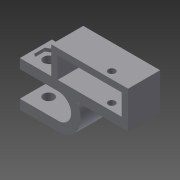
# Autodesk Inventor part: EndStopClip8mm
Saved by Autodesk Inventor 2014 SP1 (Build 180222100, 222)
## iProperties
Created: 2014-03-02
Part Number: EndStopClip8mm
Material: Generic
Document SubType Name: Modeling
Designer: Jack
Density: 1 g/cm^3
Appearance: Default
Author: Jack
Autodesk Inventor part; units mm, degrees
ref_plane "YZ Plane" through (0, 0, 0) normal (1, 0, 0) x (0, 1, 0)
ref_plane "XZ Plane" through (0, 0, 0) normal (0, 1, 0) x (-1, 0, 0)
ref_plane "XY Plane" through (0, 0, 0) normal (0, 0, 1) x (1, 0, 0)
sketch "Sketch1" plane through (0, 0, 0) normal (0, 1, 0) x (-1, 0, 0)
  arc A0 (0, 4) -> (0, -4) centre (0, 0) ccw
  line L0 (-19.8, 7.6035) -> (0, 7.6035) construction
  line L1 (0, 7.6035) -> (0, 14.0035) construction
  line L2 (0, 14.0035) -> (-19.8, 14.0035) construction
  line L3 (-19.8, 14.0035) -> (-19.8, 7.6035) construction
  line L4 (0, 7) -> (-21.8, 7)
  line L5 (0, 7) -> (12, 7)
  line L6 (12, 7) -> (12, 4)
  line L7 (12, 4) -> (5.7446, 4)
  line L8 (0, -7) -> (12, -7)
  line L9 (12, -7) -> (12, -4)
  line L10 (12, -4) -> (5.7446, -4)
  line L11 (-5.7446, 4) -> (-21.8, 4)
  line L12 (-21.8, 4) -> (-21.8, 7)
  line L13 (5.7446, 4) -> (0, 4)
  line L14 (5.7446, -4) -> (0, -4)
  arc A1 (-5.7446, 4) -> (0, -7) centre (0, 0) ccw
  dimension "d0" = 8
  dimension "d1" = 19.8
  dimension "d2" = 6.4
  dimension "d3" = 19.8
  dimension "d5" = 21.8
  dimension "d6" = 12
  dimension "d7" = 3
  dimension "d8" = 3
  dimension "d9" = 3
  dimension "d10" = 12
  dimension "d11" = 7
  dimension "d12" = 7
  dimension "d13" = 21.8
  constraints: 30 end point, 7 perpendicular, 5 parallel, 4 point on circle, 2 centre point, 2 coincident, 1 collinear, 1 horizontal, 1 tangent, 1 vertical alignment
  measures "d0" diameter of A0
  measures "d1" distance of L0.start L0.end
  measures "d2" distance of L0.end L1.end
  measures "d3" distance of L1.end L2.end
  measures "d5" distance of L4.start L4.end
  measures "d6" distance of L4.start L5.end
  measures "d7" distance of L5.end L6.end
  measures "d8" distance of L8.end L9.end
  measures "d9" distance of L11.end L4.end
  measures "d10" distance of L8.start L8.end
  measures "d11" radius of A1
  measures "d12" distance from line of point (0, 0) L4
  measures "d13" distance from line of L12 point (0, 0)
extrude "Extrusion1" add sketch "Sketch1" along normal blind 10
sketch "Sketch2" plane through (0, 0, -7) normal (0, 0, -1) x (-1, 0, 0)
  line L0 (12, 0) -> (12, 10) projected
  line L1 (0, 10) -> (12, 10) projected
  circle A0 centre (8, 5) radius 1.65
  dimension "d16" = 3.3
  dimension "d17" = 4
  dimension "d18" = 5
  constraints: 1 centre point
  measures "d16" diameter of A0
  measures "d17" distance from line of L0 A0.centre
  measures "d18" distance from line of L1 A0.centre
extrude "Extrusion2" cut sketch "Sketch2" against normal up to surface (14 mm away)
sketch "Sketch3" plane through (-12, 0, 7) normal (0, 0, 1) x (1, 0, 0)
  line L0 (0, 0) -> (33.8, 0) projected
  line L1 (33.8, 0) -> (33.8, 10) projected
  line L2 (0, 10) -> (33.8, 10) projected
  line L3 (31.8, 10) -> (31.8, 0)
  point P0 (12, 0)
  dimension "d21" = 2
  constraints: 2 end point, 2 point on line, 1 perpendicular
  measures "d21" distance between parallel lines of L1 L3
extrude "Extrusion3" add sketch "Sketch3" along normal blind 6.6
sketch "Sketch4" plane through (-12, 0, 7) normal (0, 0, 1) x (1, 0, 0)
  line L0 (31.8, 0) -> (31.8, 10) projected
  line L1 (0, 10) -> (31.8, 10) projected
  line L2 (0, 0) -> (31.8, 0) projected
  line L3 (11.8, 10) -> (11.8, 0)
  line L4 (9.8, 0) -> (9.8, 10)
  point P0 (12, 0)
  dimension "d24" = 2
  dimension "d25" = 20
  constraints: 4 end point, 4 point on line, 2 perpendicular
  measures "d24" distance between parallel lines of L3 L4
  measures "d25" distance between parallel lines of L0 L3
extrude "Extrusion4" add sketch "Sketch4" along normal blind 6.6 contours L2 L4 L1 L3
sketch "Sketch5" plane through (-12, 0, 13.6) normal (0, 0, 1) x (1, 0, 0)
  line L0 (9.8, 10) -> (9.8, 0) projected
  line L1 (33.8, 0) -> (33.8, 10) projected
  line L2 (33.8, 10) -> (31.8, 10) projected
  line L3 (31.8, 10) -> (31.8, 0) projected
  line L4 (31.8, 0) -> (33.8, 0) projected
  line L5 (9.8, 10) -> (33.8, 10)
  line L6 (33.8, 0) -> (9.8, 0)
  point P0 (12, 0)
  constraints: 4 end point, 2 parallel
extrude "Extrusion5" add sketch "Sketch5" along normal blind 2
sketch "Sketch6" plane through (-12, 0, 15.6) normal (0, 0, 1) x (1, 0, 0)
  circle A0 centre (26.5, 2.2) radius 1 projected
  circle A1 centre (26.5, 2.2) radius 1.1
  point P0 (12, 0)
  dimension "d30" = 2.2
  constraints: 1 centre point, 1 coincident
  measures "d30" diameter of A1
extrude "Extrusion6" cut sketch "Sketch6" against normal up to surface (11.6 mm away) contours A0 | A1
sketch "Sketch7" plane through (-12, 0, 7) normal (0, 0, 1) x (1, 0, 0)
  circle A0 centre (4, 5) radius 1.65 projected
  line L0 (4, 8.3486) -> (6.9, 6.6743)
  line L1 (6.9, 6.6743) -> (6.9, 3.3257)
  line L2 (6.9, 3.3257) -> (4, 1.6514)
  line L3 (4, 1.6514) -> (1.1, 3.3257)
  line L4 (1.1, 3.3257) -> (1.1, 6.6743)
  line L5 (1.1, 6.6743) -> (4, 8.3486)
  point P0 (12, 0)
  dimension "d33" = 5.8
  constraints: 12 end point, 1 coincident, 1 vertical, 13 other
  measures "d33" distance between parallel lines of L1 L4
extrude "Extrusion7" cut sketch "Sketch7" against normal blind 1
body "Solid1"
